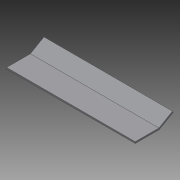
# Autodesk Inventor part: geard
Saved by Autodesk Inventor 2015 (Build 190159000, 159)
## iProperties
Created: 2015-12-11
Part Number: geard
Material: 一般
Document SubType Name: Modeling
Designer: kenta
Density: 1 g/cm^3
Appearance: 既定
Author: kenta
Autodesk Inventor part; units mm, degrees
ref_plane "YZ Plane" through (0, 0, 0) normal (1, 0, 0) x (0, 1, 0)
ref_plane "XZ Plane" through (0, 0, 0) normal (0, 1, 0) x (-1, 0, 0)
ref_plane "XY Plane" through (0, 0, 0) normal (0, 0, 1) x (1, 0, 0)
sketch "スケッチ2" plane through (0, 0, 0) normal (0, 0, 1) x (1, 0, 0)
  line L0 (0, 0) -> (80, 0)
  line L1 (80, 0) -> (80, -15)
  line L2 (80, -15) -> (0, -15)
  line L3 (0, -15) -> (0, 0)
  dimension "d4" = 80
  dimension "d5" = 15
  constraints: 8 end point, 2 parallel, 1 horizontal, 1 perpendicular
  measures "d4" distance of L1.end L2.end
  measures "d5" distance of L0.end L1.end
extrude "押し出し2" add sketch "スケッチ2" along normal blind 1
sketch "スケッチ3" plane through (80, -15, 0) normal (1, 0, 0) x (0, 0, -1)
  line L0 (0, 15) -> (-5, 23.6603)
  line L1 (0, 15) -> (10, 15) construction
  line L2 (-5, 23.6603) -> (-5.866, 23.1603)
  line L3 (-5.866, 23.1603) -> (-0.866, 14.5)
  line L4 (-0.866, 14.5) -> (0, 15)
  dimension "d8" = 10
  dimension "d9" = 120
  dimension "d10" = 1
  dimension "d11" = 10
  constraints: 10 end point, 2 perpendicular, 1 equal length, 1 horizontal
  measures "d8" distance of L0.start L0.end
  measures "d9" angle of L1 L0
  measures "d10" distance of L0.end L2.end
  measures "d11" distance of L2.end L3.end
extrude "押し出し3" add sketch "スケッチ3" against normal blind 80
